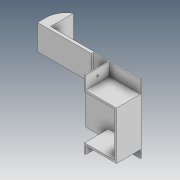
# Autodesk Inventor part: tampa 2
Saved by Autodesk Inventor 2021 (Build 250183000, 183)
## iProperties
Created: 2020-10-21
Part Number: tampa 2
Material: Genérico
Document SubType Name: Modeling
Designer: evert
Density: 1 g/cm^3
Appearance: Padrão
Author: evert
Autodesk Inventor part; units mm, degrees
ref_plane "YZ Plane" through (0, 0, 0) normal (1, 0, 0) x (0, 1, 0)
ref_plane "XZ Plane" through (0, 0, 0) normal (0, 1, 0) x (-1, 0, 0)
ref_plane "XY Plane" through (0, 0, 0) normal (0, 0, 1) x (1, 0, 0)
sketch "Esboço1" plane through (0, 0, 0) normal (0, 0, 1) x (1, 0, 0)
  line L0 (0, 0) -> (50, 0)
  line L1 (50, 0) -> (50, -31.4)
  line L2 (50, -31.4) -> (0, -31.4)
  line L3 (0, -31.4) -> (0, 0)
  dimension "d0" = 50
  dimension "d1" = 31.4
  constraints: 8 end point, 2 parallel, 1 horizontal, 1 perpendicular
  measures "d0" distance of L0.start L0.end
  measures "d1" distance of L2.end L0.start
extrude "Extrusão1" add sketch "Esboço1" along normal blind 0.5
sketch "Esboço2" plane through (0, 0, 0.5) normal (0, 0, 1) x (1, 0, 0)
  line L0 (0, -31.4) -> (50, -31.4) projected
  line L1 (50, -31.4) -> (43.6, -31.4)
  line L2 (43.6, -31.4) -> (43.6, 0)
  line L3 (50, 0) -> (0, 0) projected
  line L4 (43.6, 0) -> (50, 0)
  line L5 (50, -31.4) -> (50, 0) projected
  line L6 (50, 0) -> (50, -31.4)
  dimension "d4" = 6.4
  constraints: 8 end point, 2 point on line, 1 collinear, 1 horizontal, 1 perpendicular
  measures "d4" distance of L0.end L1.end
extrude "Extrusão2" cut sketch "Esboço2" against normal blind 0.5
sketch "Esboço3" plane through (0, 0, 0.5) normal (0, 0, 1) x (1, 0, 0)
  line L0 (0, -31.4) -> (43.6, -31.4) projected
  line L1 (43.6, -31.4) -> (13.6, -31.4)
  line L2 (13.6, -31.4) -> (13.6, -34.4)
  line L3 (13.6, -34.4) -> (43.6, -34.4)
  line L4 (43.6, -34.4) -> (43.6, -31.4)
  point P0 (0, 0)
  dimension "d7" = 30
  dimension "d8" = 3
  constraints: 8 end point, 2 parallel, 1 horizontal, 1 perpendicular
  measures "d7" distance of L3.end L2.end
  measures "d8" distance of L3.end L0.end
extrude "Extrusão3" add sketch "Esboço3" against normal blind 0.5
sketch "Esboço4" plane through (0, 0, 0.5) normal (0, 0, 1) x (1, 0, 0)
  line L0 (43.6, -34.4) -> (43.6, 0) projected
  line L1 (43.6, -34.4) -> (44.6, -34.4)
  line L2 (44.6, -34.4) -> (44.6, 0)
  line L3 (44.6, 0) -> (43.6, 0)
  line L4 (43.6, 0) -> (43.6, -34.4)
  point P0 (0, 0)
  dimension "d11" = 1
  constraints: 8 end point, 2 parallel, 1 horizontal, 1 perpendicular
  measures "d11" distance of L3.end L2.end
extrude "Extrusão4" add sketch "Esboço4" against normal blind 0.5
sketch "Esboço5" plane through (0, 0, 0.5) normal (0, 0, 1) x (1, 0, 0)
  line L0 (44.6, -34.4) -> (13.6, -34.4) projected
  line L1 (44.6, -34.4) -> (44.6, -29.5)
  line L2 (44.6, 0) -> (44.6, -34.4) projected
  line L3 (44.6, 0) -> (44.6, -7.4)
  line L4 (44.6, -7.4) -> (29.6, -7.4)
  line L5 (44.6, -29.5) -> (29.6, -29.5)
  line L6 (29.6, -29.5) -> (29.6, -30.5)
  line L7 (29.6, -30.5) -> (44.6, -30.5)
  line L8 (29.6, -7.4) -> (29.6, -6.4)
  line L9 (29.6, -6.4) -> (44.6, -6.4)
  line L10 (44.6, -7.4) -> (44.6, -6.4)
  line L11 (29.6, -6.4) -> (30.1, -6.4)
  line L12 (30.1, -6.4) -> (30.1, 0)
  line L13 (44.6, 0) -> (0, 0) projected
  line L14 (29.6, 0) -> (29.6, -6.4)
  line L15 (29.6, -30.5) -> (29.6, -34.4)
  line L16 (30.1, -30.5) -> (30.1, -34.4)
  line L17 (29.6, -34.4) -> (30.1, -34.4)
  dimension "d14" = 4.9
  dimension "d15" = 7.4
  dimension "d16" = 15
  dimension "d17" = 15
  dimension "d18" = 1
  dimension "d19" = 1
  dimension "d20" = 0.5
  constraints: 30 end point, 12 point on line, 5 perpendicular, 2 horizontal, 1 parallel, 1 vertical
  measures "d14" distance of L0.start L1.end
  measures "d15" distance of L2.start L3.end
  measures "d16" distance of L3.end L4.end
  measures "d17" distance of L1.end L5.end
  measures "d18" distance of L5.end L6.end
  measures "d19" distance of L4.end L8.end
  measures "d20" distance of L8.end L11.end
extrude "Extrusão5" add sketch "Esboço5" along normal blind 12 contours L0 L15 L7 L16 | L7 L6 L5 L1 | L2 L4 L8 L9 | L12 L9 L14 L13
sketch "Esboço6" plane through (0, 0, 0.5) normal (0, 0, 1) x (1, 0, 0)
  line L0 (44.6, -34.4) -> (44.6, -30.5) projected
  line L1 (44.6, -34.4) -> (45.6, -34.4)
  line L2 (45.6, -34.4) -> (45.6, 0)
  line L3 (45.6, 0) -> (44.6, 0)
  line L4 (44.6, 0) -> (44.6, -34.4)
  point P0 (0, 0)
  dimension "d23" = 1
  constraints: 8 end point, 2 parallel, 1 horizontal, 1 perpendicular
  measures "d23" distance of L3.end L2.end
extrude "Extrusão6" add sketch "Esboço6" against normal blind 0.5
sketch "Esboço7" plane through (0, 0, 0.5) normal (0, 0, 1) x (1, 0, 0)
  line L0 (44.6, -30.5) -> (30.1, -30.5) projected
  line L1 (44.6, -30.5) -> (45.6, -30.5)
  line L2 (45.6, -34.4) -> (45.6, 0) projected
  line L3 (45.6, -30.5) -> (45.6, -6.4)
  line L4 (30.1, -6.4) -> (44.6, -6.4) projected
  line L5 (44.6, -6.4) -> (45.6, -6.4)
  line L6 (44.6, -6.4) -> (44.6, -30.5)
  point P0 (0, 0)
  constraints: 8 end point, 2 horizontal, 1 perpendicular, 1 point on line, 1 vertical
extrude "Extrusão7" add sketch "Esboço7" along normal blind 12
sketch "Esboço8" plane through (0, 0, 0.5) normal (0, 0, 1) x (1, 0, 0)
  line L0 (29.6, -29.5) -> (29.6, -34.4) projected
  line L1 (29.6, -31.7209) -> (18.1, -31.7209)
  line L2 (18.1, -34.4) -> (18.1, -31.7209)
  line L3 (18.1, -31.7209) -> (18.1, -12.7)
  line L4 (18.1, -12.7) -> (0, -12.7)
  line L5 (0, 0) -> (0, -31.4) projected
  line L6 (18.1, -34.4) -> (0, -34.4)
  line L7 (0, -34.4) -> (0, -12.7)
  dimension "d28" = 11.5
  constraints: 12 end point, 3 point on line, 2 horizontal, 1 collinear, 1 perpendicular, 1 vertical
  measures "d28" distance of L1.start L1.end
extrude "Extrusão8" cut sketch "Esboço8" against normal blind 12
sketch "Esboço9" plane through (0, 0, 0.5) normal (0, 0, 1) x (1, 0, 0)
  line L0 (0, 0) -> (0, -12.7) projected
  line L1 (0, 0) -> (-5, 0)
  line L2 (-5, 0) -> (-5, -12.7)
  line L3 (-5, -12.7) -> (0, -12.7)
  line L4 (0, -12.7) -> (0, 0)
  dimension "d31" = 5
  constraints: 8 end point, 2 parallel, 1 horizontal, 1 perpendicular
  measures "d31" distance of L3.end L2.end
extrude "Extrusão9" add sketch "Esboço9" against normal blind 12
fillet "Arredondamento1" radius 10 1 edges at (-5, -6.35, -11.5)
sketch "Esboço10" plane through (0, 0, 0.5) normal (0, 0, 1) x (1, 0, 0)
  line L0 (-5, 0) -> (-5, -12.7) projected
  line L1 (-5, 0) -> (22, 0)
  line L2 (22, 0) -> (22, -12.7)
  line L3 (22, -12.7) -> (-5, -12.7)
  line L4 (-5, -12.7) -> (-5, 0)
  point P0 (0, 0)
  dimension "d37" = 27
  constraints: 8 end point, 2 parallel, 1 horizontal, 1 perpendicular
  measures "d37" distance of L0.start L1.end
extrude "Extrusão10" add sketch "Esboço10" along normal blind 1
sketch "Esboço11" plane through (30.1, -6.4, 0.5) normal (1, 0, 0) x (0, 0, -1)
  line L0 (0, 6.4) -> (-12, 6.4) projected
  line L1 (-12, 6.4) -> (-6, 6.4)
  line L2 (-6, 6.4) -> (-6, -28)
  line L3 (0, -28) -> (-12, -28) projected
  line L4 (-6, 6.4) -> (-6, 3.2)
  line L5 (-6, -28) -> (-6, -26.1)
  circle A0 centre (-6, -26.1) radius 0.5
  circle A1 centre (-6, 3.2) radius 0.5
  point P0 (0.5, 6.4)
  dimension "d38" = 3.2
  dimension "d39" = 1.9
  dimension "d40" = 1
  dimension "d41" = 1
  constraints: 8 end point, 2 centre point, 2 coincident, 2 midpoint, 2 point on line
  measures "d38" distance of L1.end L4.end
  measures "d39" distance of L2.end L5.end
  measures "d40" diameter of A0
  measures "d41" diameter of A1
extrude "Extrusão11" cut sketch "Esboço11" against normal blind 1
